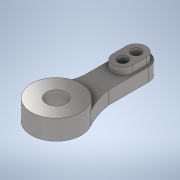
# Autodesk Inventor part: ServoArm
Saved by Autodesk Inventor 2020 (Build 240168000, 168)
## iProperties
Created: 2023-12-24
Part Number: ServoArm
Material: Stainless Steel
Document SubType Name: Modeling
Designer: smz3rm
Mass: 4 g
Surface Area: 12.9711 cm^2
Volume: 1.54175 cm^3
Density: 2.59446 g/cm^3
Appearance: Semi-Polished
Author: smz3rm
Autodesk Inventor part; units mm, degrees
ref_plane "YZ Plane" through (0, 0, 0) normal (1, 0, 0) x (0, 1, 0)
ref_plane "XZ Plane" through (0, 0, 0) normal (0, 1, 0) x (-1, 0, 0)
ref_plane "XY Plane" through (0, 0, 0) normal (0, 0, 1) x (1, 0, 0)
sketch "Sketch1" plane through (0, 0, 0) normal (0, 1, 0) x (-1, 0, 0)
  circle A0 centre (0, 0) radius 7.5
  line L0 (0, 0) -> (0, -24) construction
  line L1 (-3.75, 0) -> (-3.75, -24)
  line L2 (3.75, -24) -> (3.75, 0)
  arc A1 (3.75, 0) -> (-3.75, 0) centre (0, 0) ccw
  arc A2 (-3.75, -24) -> (3.75, -24) centre (0, -24) ccw
  arc A3 (6.5919, -3.5773) -> (3.75, -12) centre (29.4438, -15.9785) ccw
  line L3 (0, -34.8) -> (0, 14.55) projected
  arc A4 (-3.75, -12) -> (-6.5919, -3.5773) centre (-29.4438, -15.9785) ccw
  circle A5 centre (0, -24) radius 1.5
  circle A6 centre (0, -20) radius 1.5
  point P0 (0, -12)
  point P1 (-6.5919, -3.5773)
  point P2 (-3.75, -12)
  dimension "d0" = 15
  dimension "d1" = 24
  dimension "d2" = 7.5
  dimension "d3" = 26
  dimension "d4" = 3
  dimension "d5" = 3
  dimension "d6" = 20
  constraints: 8 end point, 8 point on circle, 6 centre point, 4 tangent, 3 symmetric about line, 2 coincident, 2 midpoint, 1 parallel, 1 point on line, 1 vertical, 5 other
  measures "d1" distance of L0.start L0.end
  measures "d2" diameter of A2
  measures "d3" radius of A3
  measures "d4" diameter of A5
  measures "d5" diameter of A6
  measures "d6" distance of point (0, 0) A6.centre
extrude "Extrusion1" add sketch "Sketch1" along normal blind 6 contours A0 L2 A1 L3 | A3 L2 A0 | L2 A2 L3 A5 A6 A0 | A0 L3 A1 L2 | L3 A1 L1 A0 | L3 A6 A5 A2 L1 A0 | A0 L1 A1 L3 | A0 L1 A4
sketch "Sketch2" plane through (0, 6, 0) normal (0, 1, 0) x (1, 0, 0)
  circle A0 centre (0, 0) radius 7.5
  arc A1 (-6.5919, 3.5773) -> (6.5919, 3.5773) centre (0, 0) ccw projected
  circle A2 centre (0, 20) radius 1.5 projected
  circle A3 centre (0, 24) radius 1.5 projected
  circle A4 centre (0, 24) radius 1.5 projected
  line L0 (0, 20) -> (0, 24) construction
  line L1 (3, 20) -> (3, 24)
  line L2 (-3, 24) -> (-3, 20)
  arc A5 (-3, 20) -> (3, 20) centre (0, 20) ccw
  arc A6 (3, 24) -> (-3, 24) centre (0, 24) ccw
  arc A7 (-6.5919, 3.5773) -> (6.5919, 3.5773) centre (0, 0) ccw projected
  arc A8 (3.75, 12) -> (6.5919, 3.5773) centre (29.4438, 15.9785) ccw projected
  line L3 (3.75, 12) -> (3.75, 24) projected
  arc A9 (3.75, 24) -> (-3.75, 24) centre (0, 24) ccw projected
  line L4 (-3.75, 24) -> (-3.75, 12) projected
  arc A10 (-6.5919, 3.5773) -> (-3.75, 12) centre (-29.4438, 15.9785) ccw projected
  circle A11 centre (0, 20) radius 1.5 projected
  circle A12 centre (0, 24) radius 1.5 projected
  point P0 (0, 22)
  point P1 (-6.5919, 3.5773)
  point P2 (6.5919, 3.5773)
  dimension "d9" = 6
  constraints: 8 end point, 4 point on circle, 4 tangent, 3 centre point, 2 concentric, 1 coincident, 1 midpoint, 1 parallel, 1 vertical
  measures "d9" diameter of A6
extrude "Extrusion2" cut sketch "Sketch2" against normal blind 2 contours A0 A10 L4 A9 L3 A8
sketch "Sketch3" plane through (0, 6, 0) normal (0, 1, 0) x (1, 0, 0)
  circle A0 centre (0, 0) radius 3
  dimension "d12" = 6
  constraints: 1 centre point, 1 coincident
  measures "d12" diameter of A0
extrude "Extrusion3" cut sketch "Sketch3" against normal through all
body "Solid1"
